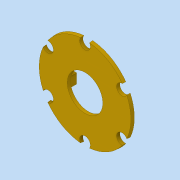
# Autodesk Inventor part: aftServoAssemblyForwardDisc
Saved by Autodesk Inventor 2017 (Build 210142000, 142)
## iProperties
Created: 2016-10-06
Part Number: aftServoAssemblyForwardDisc
Material: Generic
Document SubType Name: Modeling
Designer: techn
Density: 1 g/cm^3
Appearance: Gold
Author: techn
Autodesk Inventor part; units mm, degrees
ref_plane "YZ Plane" through (0, 0, 0) normal (1, 0, 0) x (0, 1, 0)
ref_plane "XZ Plane" through (0, 0, 0) normal (0, 1, 0) x (-1, 0, 0)
sketch "Sketch1" plane through (0, 0, 0) normal (0, 0, 1) x (1, 0, 0)
  circle A0 centre (0, 0) radius 50.8
  dimension "d0" = 101.6
  constraints: 1 centre point, 1 coincident
  measures "d0" diameter of A0
ref_plane "Work Plane1" through (0, 0, 279.4) normal (0, 0, 1) x (1, 0, 0)
sketch "Sketch2" plane through (0, 0, 279.4) normal (0, 0, 1) x (1, 0, 0)
  circle A0 centre (0, 0) radius 7.1437
  dimension "d3" = 14.2875
  constraints: 1 centre point, 1 coincident
  measures "d3" diameter of A0
loft "Loft2" add profiles "Sketch1", "Sketch2"
sketch "Sketch15" plane through (0, 0, 0) normal (0, 1, 0) x (-1, 0, 0)
  line L0 (-7.1437, 279.4) -> (7.1437, 279.4) projected
  line L1 (0, 279.4) -> (-7.1437, 279.4)
  line L2 (-50.8, 0) -> (50.8, 0) projected
  line L3 (50.8, 0) -> (-50.8, 0)
  line L4 (-50.8, 0) -> (-50.8, 279.4)
  line L5 (-50.8, 279.4) -> (50.8, 279.4)
  line L6 (50.8, 279.4) -> (50.8, 0)
  line L7 (-7.1437, 279.4) -> (0, 302.26)
  line L8 (0, 279.4) -> (0, 88.9)
  line L9 (0, 88.9) -> (-46.3803, 88.9)
  line L10 (0, 0) -> (-50.8, 0)
  line L11 (0, 88.9) -> (0, 0)
  line L12 (0, 84.1375) -> (-46.8411, 84.1375)
  line L13 (0, 68.2625) -> (-48.1941, 68.2625)
  line L14 (-48.1941, 68.2625) -> (-45.0191, 68.2625)
  line L15 (-45.0191, 68.2625) -> (-45.0191, 65.0875)
  line L16 (-45.0191, 65.0875) -> (-45.2731, 65.0875)
  line L17 (-45.2731, 65.0875) -> (-45.0191, 68.2625)
  line L18 (-45.2731, 65.0875) -> (0, 65.0875)
  point P0 (0, 0)
  dimension "d258" = 190.5
  dimension "d259" = 88.9
  dimension "d264" = 4.7625
  dimension "d315" = 3.175
  dimension "d316" = 3.175
  dimension "d317" = 0.254
  dimension "d330" = 15.875
  constraints: 34 end point, 4 horizontal, 4 parallel, 4 point on line, 3 perpendicular, 2 vertical, 1 midpoint, 6 other
  measures "d258" distance of L1.start L8.end
  measures "d259" distance between parallel lines of L10 L9
  measures "d264" distance between parallel lines of L12 L9
  measures "d315" distance of L13.end L14.end
  measures "d316" distance of L14.end L15.end
  measures "d317" distance of L15.end L16.end
  measures "d330" distance between parallel lines of L13 L12
extrude "Extrusion37" cut sketch "Sketch15" along normal through all both and the other way through all
revolve "Revolution11" add sketch "Sketch15" angle 360 about axis through (0, 0, 88.9) along (0, 0, -1) contours L11 L18 L15 L13 | L15 L16 L17
sketch "Sketch59" plane through (0, 0, 68.2625) normal (0, 0, 1) x (1, 0, 0)
  line L0 (0, 0) -> (0, 41.91)
  circle A0 centre (0, 41.91) radius 5.334
  circle A1 centre (-36.2951, 20.955) radius 5.334
  circle A2 centre (-36.2951, -20.955) radius 5.334
  circle A3 centre (0, -41.91) radius 5.334
  circle A4 centre (36.2951, -20.955) radius 5.334
  circle A5 centre (36.2951, 20.955) radius 5.334
  dimension "d319" = 41.91
  dimension "d320" = 10.668
  dimension "d323" = 360
  constraints: 6 centre point, 2 end point, 1 coincident, 1 vertical, 13 other
  measures "d319" distance of L0.start L0.end
  measures "d320" diameter of A0
extrude "Extrusion45" cut sketch "Sketch59" against normal blind 25.4
sketch "Sketch60" plane through (0, -41.91, 65.0875) normal (0, 0, -1) x (-1, 0, 0)
  circle A0 centre (0, 41.91) radius 17.5
  point P0 (0, 41.91)
  dimension "d327" = 35
  constraints: 1 centre point, 1 coincident
  measures "d327" diameter of A0
extrude "Extrusion46" cut sketch "Sketch60" against normal blind 25.4
sketch "Sketch61" plane through (0, -41.91, 65.0875) normal (0, 0, -1) x (-1, 0, 0)
  line L0 (18, 45.085) -> (37.05, 45.085)
  line L1 (37.05, 45.085) -> (37.05, 35.56)
  line L2 (37.05, 35.56) -> (18, 35.56)
  line L3 (18, 35.56) -> (18, 45.085)
  line L4 (0, 41.91) -> (0, -3.2701)
  line L5 (-18, 45.085) -> (-37.05, 45.085)
  line L6 (-37.05, 45.085) -> (-37.05, 35.56)
  line L7 (-37.05, 35.56) -> (-18, 35.56)
  line L8 (-18, 35.56) -> (-18, 45.085)
  dimension "d331" = 19.05
  dimension "d332" = 9.525
  dimension "d333" = 18
  dimension "d347" = 3.175
  constraints: 18 end point, 4 symmetric about line, 2 parallel, 1 horizontal, 1 perpendicular, 1 vertical
  measures "d331" distance of L1.end L2.end
  measures "d332" distance of L0.end L1.end
  measures "d333" horizontal distance of L2.end L4.start
  measures "d347" distance from line of L0 L4.start
extrude "Extrusion47" add sketch "Sketch61" along normal blind 6.604
sketch "Sketch62" plane through (18, 3.175, 65.0875) normal (0, 1, 0) x (1, 0, 0)
  line L0 (-23.334, 0) -> (-12.666, 0) projected
  line L1 (-18, 0) -> (-18, 51.1143)
  line L2 (19.05, 0) -> (0, 0) projected
  line L3 (19.05, 0) -> (19.05, 6.604) projected
  line L4 (0, 6.604) -> (19.05, 6.604) projected
  line L5 (0, 0) -> (0, 6.604) projected
  circle A0 centre (14.605, 2.794) radius 1.27
  circle A1 centre (4.445, 2.794) radius 1.27
  line L6 (19.05, 6.604) -> (0, 6.604) projected
  line L7 (9.525, 6.604) -> (9.525, 11.5709)
  circle A2 centre (-50.605, 2.794) radius 1.27
  circle A3 centre (-40.445, 2.794) radius 1.27
  point P0 (-18, 65.0875)
  point P1 (-22.2982, 0)
  point P2 (-13.7018, 0)
  dimension "d337" = 2.54
  dimension "d338" = 2.54
  dimension "d339" = 10.16
  dimension "d342" = 5.08
  dimension "d345" = 3.81
  dimension "d346" = 3.81
  constraints: 4 centre point, 4 end point, 2 midpoint, 2 symmetric about line, 2 vertical, 2 other
  measures "d337" diameter of A0
  measures "d338" diameter of A1
  measures "d339" distance of A0.centre A1.centre
  measures "d342" distance from line of L7 A1.centre
  measures "d345" distance from line of L4 A1.centre
  measures "d346" distance from line of L4 A0.centre
extrude "Extrusion48" cut sketch "Sketch62" against normal through all contours A0 | A1 | A2 | A3
body "Solid2"
